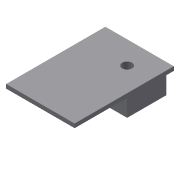
# Autodesk Inventor part: LG_G2_Lens
Saved by Autodesk Inventor 2019 (Build 230136000, 136)
## iProperties
Created: 2017-06-16
Part Number: LG_G2_Lens
Material: Generisch
Document SubType Name: Modeling
Designer: diederichbenedict
Density: 1 g/cm^3
Appearance: Vorgabe
Author: diederichbenedict
Autodesk Inventor part; units mm, degrees
ref_plane "YZ Plane" through (0, 0, 0) normal (1, 0, 0) x (0, 1, 0)
ref_plane "XZ Plane" through (0, 0, 0) normal (0, 1, 0) x (-1, 0, 0)
ref_plane "XY Plane" through (0, 0, 0) normal (0, 0, 1) x (1, 0, 0)
sketch "Skizze1" plane through (0, 0, 0) normal (0, 0, 1) x (1, 0, 0)
  line L0 (-4.85, 4.85) -> (4.85, 4.85)
  line L1 (4.85, 4.85) -> (4.85, -4.85)
  line L2 (4.85, -4.85) -> (-4.85, -4.85)
  line L3 (-4.85, -4.85) -> (-4.85, 4.85)
  line L4 (-4.85, 4.85) -> (4.85, -4.85) construction
  line L5 (4.85, 4.85) -> (-4.85, -4.85) construction
  circle A0 centre (0, 0) radius 1.2261
  dimension "d0" = 9.7
  dimension "d1" = 9.7
  constraints: 12 end point, 2 midpoint, 2 parallel, 1 centre point, 1 coincident, 1 horizontal, 1 perpendicular
  measures "d0" distance of L1.end L2.end
  measures "d1" distance of L0.end L1.end
extrude "Extrusion1" add sketch "Skizze1" along normal blind 5.4
sketch "Sketch2" plane through (0, 0, 5.4) normal (0, 0, 1) x (1, 0, 0)
  circle A0 centre (0, 0) radius 1.2261 projected
  line L0 (4.85, 4.85) -> (-4.85, 4.85) projected
  line L1 (-4.85, 4.85) -> (-4.85, -4.85) projected
  line L2 (-4.85, -4.85) -> (4.85, -4.85) projected
  line L3 (4.85, -4.85) -> (4.85, 4.85) projected
  line L4 (-11.05, 5.65) -> (5.95, 5.65)
  line L5 (5.95, 5.65) -> (5.95, -18.9856)
  line L6 (5.95, -18.9856) -> (-11.05, -18.9856)
  line L7 (-11.05, -18.9856) -> (-11.05, 5.65)
  dimension "d4" = 10.8
  dimension "d5" = 15.9
  dimension "d6" = 10.5
  constraints: 8 end point, 2 parallel, 1 horizontal, 1 perpendicular
  measures "d4" distance between parallel lines of L5 L1
  measures "d5" distance between parallel lines of L7 L3
  measures "d6" distance between parallel lines of L2 L4
extrude "Extrusion2" add sketch "Sketch2" along normal blind 1 contours L3 L2 L1 L0 | L4 L5 L6 L7
